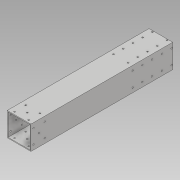
# Autodesk Inventor part: square_tube_2
Saved by Autodesk Inventor 2017 (Build 210142000, 142)
## iProperties
Part Number: square_tube_2
Material: Aluminium 6061
Document SubType Name: Modeling
Designer: Max
Mass: 424.198 g
Surface Area: 1592.96 cm^2
Volume: 157.11 cm^3
Density: 2.7 g/cm^3
Appearance: Vorgabe
Author: Max
Autodesk Inventor part; units mm, degrees
note: some values were not read from the file. Chosen so that the rebuilt part matches the saved one: direction of "Bohrung1".
ref_plane "YZ Plane" through (0, 0, 0) normal (1, 0, 0) x (0, 1, 0)
ref_plane "XZ Plane" through (0, 0, 0) normal (0, 1, 0) x (-1, 0, 0)
sketch "Skizze1" plane through (0, 0, 0) normal (0, 1, 0) x (-1, 0, 0)
  line L0 (-29.25, 29.25) -> (29.25, 29.25)
  line L1 (29.25, 29.25) -> (29.25, -29.25)
  line L2 (29.25, -29.25) -> (-29.25, -29.25)
  line L3 (-29.25, -29.25) -> (-29.25, 29.25)
  line L4 (-29.25, 29.25) -> (29.25, -29.25) construction
  line L5 (29.25, 29.25) -> (-29.25, -29.25) construction
  line L6 (27.25, -27.25) -> (27.25, 27.25)
  line L7 (27.25, 27.25) -> (-27.25, 27.25)
  line L8 (-27.25, 27.25) -> (-27.25, -27.25)
  line L9 (-27.25, -27.25) -> (27.25, -27.25)
  point P0 (0, 0)
  dimension "d0" = 2
  dimension "d1" = 54.5
  dimension "d2" = 54.5
  constraints: 20 end point, 4 parallel, 2 midpoint, 2 perpendicular, 1 horizontal, 3 other
  measures "d0" distance between parallel lines of L6 L1
  measures "d1" distance of L6.start L6.end
  measures "d2" distance of L8.end L6.start
extrude "Extrusion1" add sketch "Skizze1" along normal blind 350
sketch "Skizze2" plane through (-29.25, 0, 29.25) normal (0, 0, 1) x (1, 0, 0)
  line L0 (11.75, 6.25) -> (46.75, 6.25)
  line L1 (46.75, 6.25) -> (46.75, 33.75)
  line L2 (46.75, 33.75) -> (11.75, 33.75)
  line L3 (11.75, 33.75) -> (11.75, 6.25)
  line L4 (11.75, 6.25) -> (46.75, 33.75) construction
  line L5 (46.75, 6.25) -> (11.75, 33.75) construction
  line L6 (58.5, 0) -> (0, 0) projected
  line L7 (58.5, 0) -> (58.5, 350) projected
  line L8 (0, 350) -> (58.5, 350) projected
  line L9 (0, 0) -> (0, 350) projected
  point P0 (29.25, 0)
  point P1 (29.25, 20)
  dimension "d5" = 35
  dimension "d6" = 27.5
  dimension "d7" = 58.5
  dimension "d8" = 29.25
  dimension "d42" = 20
  constraints: 12 end point, 2 midpoint, 2 parallel, 1 horizontal, 1 perpendicular
  measures "d5" distance of L1.end L2.end
  measures "d6" distance of L0.end L1.end
  measures "d7" distance of L6.start L6.end
  measures "d8" distance from line of point (29.25, 20) L9
  measures "d42" distance from line of L6 point (29.25, 20)
hole "Bohrung1" at (0, 20, 29.25) at (-17.5, 6.25, 29.25) at (-17.5, 33.75, 29.25) at (17.5, 6.25, 29.25) at (17.5, 33.75, 29.25) direction (0, 0, -1) diameter 3.4 end up to surface clearance for "Inbusschraube ISO 4762" size "M3" standard "ISO"
mirror "Spiegeln1" about plane through (0, 0, 0) normal (0, 0, 1) of "Bohrung1"
ref_plane "Arbeitsebene2" through (0, 175, 0) normal (0, -1, 0) x (1, 0, 0)
pattern_circular "Runde Anordnung1" count 2 over 90 about axis through (0, -10, 0) along (0, 1, 0) of "Bohrung1", "Spiegeln1"
sketch "Skizze4" plane through (-29.25, 0, 29.25) normal (0, 0, 1) x (1, 0, 0)
  circle A0 centre (46.75, 6.25) radius 1.7 projected
  circle A1 centre (11.75, 6.25) radius 1.7 projected
  circle A2 centre (29.25, 20) radius 1.7 projected
  circle A3 centre (11.75, 33.75) radius 1.7 projected
  circle A4 centre (46.75, 33.75) radius 1.7 projected
  line L0 (58.5, 0) -> (0, 0) projected
  line L1 (58.5, 0) -> (58.5, 350) projected
  line L2 (0, 350) -> (58.5, 350) projected
  line L3 (0, 0) -> (0, 350) projected
  point P0 (29.25, 0)
  point P1 (11.25, 347)
  point P2 (47.25, 347)
  dimension "d25" = 36
  dimension "d26" = 58.5
  dimension "d27" = 11.25
  dimension "d28" = 3
  measures "d25" distance of point (47.25, 347) point (11.25, 347)
  measures "d26" distance of L2.start L1.end
  measures "d27" distance from line of point (11.25, 347) L3
  measures "d28" distance from line of L2 point (11.25, 347)
hole "Bohrung2" at (-18, 347, 29.25) at (18, 347, 29.25) direction (0, 0, -1) diameter 3.4 end through all clearance for "Inbusschraube ISO 4762" size "M3" standard "ISO"
pattern_linear "Rechteckige Anordnung1" count 5 spacing 24 along (0, -1, 0) of "Bohrung2"
pattern_circular "Runde Anordnung2" count 2 over 90 about axis through (0, -10, 0) along (0, 1, 0) of "Bohrung2", "Rechteckige Anordnung1"
ref_plane "Arbeitsebene1" through (0, 0, 0) normal (0, 0, 1) x (1, 0, 0)
ref_plane "Arbeitsebene5" through (0, 0, 0) normal (1, 0, 0) x (0, 0, -1)
ref_plane "Arbeitsebene6" through (0, 0, 0) normal (1, 0, 0) x (0, 0, -1)
equation "\"d8\" = 0.5 * d7"
equation "\"d27\" = -0.5 * d25 + 0.5 * d26"
